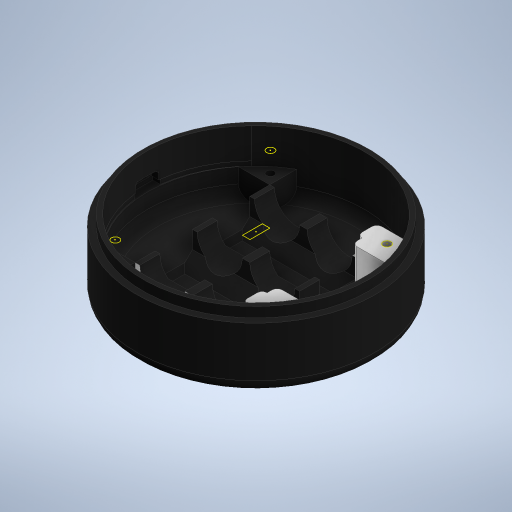
# Autodesk Inventor part: Socle test mesure
Saved by Autodesk Inventor 2024 (Build 280153000, 153)
## iProperties
Created: 2025-01-19
Part Number: Socle test mesure
Material: Générique
Document SubType Name: Modeling
Designer: malam
Density: 1 g/cm^3
Appearance: Par défaut
Author: malam
Autodesk Inventor part; units mm, degrees
ref_plane "YZ Plane" through (0, 0, 0) normal (1, 0, 0) x (0, 1, 0)
ref_plane "XZ Plane" through (0, 0, 0) normal (0, 1, 0) x (-1, 0, 0)
ref_plane "XY Plane" through (0, 0, 0) normal (0, 0, 1) x (1, 0, 0)
sketch "Esquisse1" plane through (0, 0, 0) normal (0, 1, 0) x (-1, 0, 0)
  circle A0 centre (0, 0) radius 45.31
  circle A1 centre (0, 0) radius 47.89
  line L0 (19.5, -32.55) -> (1.5, -32.55)
  line L1 (1.5, -32.55) -> (1.5, 32.55)
  line L2 (1.5, 32.55) -> (19.5, 32.55)
  line L3 (19.5, 32.55) -> (19.5, -32.55)
  line L4 (-1.5, -32.55) -> (-19.5, -32.55)
  line L5 (-19.5, -32.55) -> (-19.5, 32.55)
  line L6 (-19.5, 32.55) -> (-1.5, 32.55)
  line L7 (-1.5, 32.55) -> (-1.5, -32.55)
  line L8 (19.5, -32.55) -> (-19.5, 32.55) construction
  line L9 (19.5, 32.55) -> (-19.5, -32.55) construction
  line L10 (19.5, -32.55) -> (19.5, -43.7402)
  line L11 (19.5, 32.55) -> (19.5, 43.7402)
  point P0 (0, 0)
  point P1 (0, 0)
  dimension "d0" = 90.62
  dimension "d11" = 2.58
  dimension "d16" = 18
  dimension "d17" = 65.1
  dimension "d18" = 18
  dimension "d19" = 3
  constraints: 24 end point, 4 parallel, 2 centre point, 2 horizontal, 2 perpendicular, 2 point on circle, 1 midpoint, 1 point on line, 1 vertical
  measures "d0" diameter of A0
  measures "d11" radial gap between concentric circles of A0 A1
  measures "d16" distance of L1.end L3.start
  measures "d17" distance of L0.end L1.end
  measures "d18" distance of L5.end L7.start
  measures "d19" distance between parallel lines of L7 L1
extrude "Extrusion1" add sketch "Esquisse1" along normal blind 20 contours A0 L11 A1 L10 | A0 L10 A1 L11
sketch "Esquisse4" plane through (0, 0, 0) normal (0, -1, 0) x (1, 0, 0)
  circle A0 centre (0, 0) radius 47.89 projected
  circle A1 centre (0, 0) radius 45.31 projected
extrude "Extrusion4" add sketch "Esquisse4" against normal blind 5 contours A1
fillet "Congé2" radius 5 1 edges at (47.89, 0, 0)
sketch "Esquisse6" plane through (0, 5, 0) normal (0, 1, 0) x (1, 0, 0)
  line L0 (19.5, 32.55) -> (19.5, -32.55) projected
  line L1 (1.5, -32.55) -> (1.5, 32.55) projected
  line L2 (-1.5, 32.55) -> (-1.5, -32.55) projected
  line L3 (-19.5, -32.55) -> (-19.5, 32.55) projected
  line L4 (-19.5, 32.55) -> (-1.5, 32.55) projected
  line L5 (1.5, 32.55) -> (19.5, 32.55) projected
  line L6 (19.5, -32.55) -> (1.5, -32.55) projected
  line L7 (-1.5, -32.55) -> (-19.5, -32.55) projected
  point P0 (0, 0)
sketch "Esquisse7" plane through (0, 20, 0) normal (0, 1, 0) x (1, 0, 0)
  circle A0 centre (0, 0) radius 45.155
  circle A1 centre (0, 0) radius 43.5
  circle A2 centre (0, 0) radius 47.89 projected
  circle A3 centre (0, 0) radius 45.31 projected
  dimension "d35" = 90.31
  dimension "d36" = 87
  constraints: 2 centre point, 2 coincident
  measures "d35" diameter of A0
  measures "d36" diameter of A1
extrude "Extrusion5" add sketch "Esquisse7" against normal up to surface (15 mm away) contours A0 | A3
extrude "Extrusion6" add sketch "Esquisse7" along normal blind 4 contours A0 | A3
ref_plane "Plan de construction1" through (0, 5, 0) normal (0, 1, 0) x (1, 0, 0)
sketch "Esquisse8" plane through (0, 5, 0) normal (0, 1, 0) x (1, 0, 0)
  line L0 (-21.5, -4) -> (21.5, -4)
  line L1 (21.5, -4) -> (21.5, 4)
  line L2 (21.5, 4) -> (-21.5, 4)
  line L3 (-21.5, 4) -> (-21.5, -4)
  line L4 (-21.5, -4) -> (21.5, 4) construction
  line L5 (21.5, -4) -> (-21.5, 4) construction
  line L6 (-21.5, 19) -> (21.5, 19)
  line L7 (21.5, 19) -> (21.5, 27)
  line L8 (21.5, 27) -> (-21.5, 27)
  line L9 (-21.5, 27) -> (-21.5, 19)
  line L10 (-21.5, 19) -> (21.5, 27) construction
  line L11 (21.5, 19) -> (-21.5, 27) construction
  line L12 (-21.5, -27) -> (21.5, -27)
  line L13 (21.5, -27) -> (21.5, -19)
  line L14 (21.5, -19) -> (-21.5, -19)
  line L15 (-21.5, -19) -> (-21.5, -27)
  line L16 (-21.5, -27) -> (21.5, -19) construction
  line L17 (21.5, -27) -> (-21.5, -19) construction
  point P0 (0, 0)
  point P1 (0, 23)
  point P2 (0, -23)
  dimension "d42" = 43
  dimension "d43" = 8
  dimension "d44" = 43
  dimension "d45" = 8
  dimension "d46" = 43
  dimension "d47" = 8
  dimension "d48" = 15
  dimension "d49" = 15
  constraints: 36 end point, 6 midpoint, 6 parallel, 3 horizontal, 3 perpendicular, 2 collinear
  measures "d42" distance of L2.end L1.end
  measures "d43" distance of L0.end L1.end
  measures "d44" distance of L8.end L7.end
  measures "d45" distance of L6.end L7.end
  measures "d46" distance of L14.end L13.end
  measures "d47" distance of L12.end L13.end
  measures "d48" distance between parallel lines of L2 L6
  measures "d49" distance between parallel lines of L14 L0
extrude "Extrusion7" add sketch "Esquisse8" along normal blind 10
sketch "Esquisse9" plane through (-21.5, 5, 27) normal (0, 0, 1) x (1, 0, 0)
  line L0 (43, 0) -> (0, 0) projected
  line L1 (43, 0) -> (43, 10) projected
  line L2 (0, 10) -> (43, 10) projected
  line L3 (0, 0) -> (0, 10) projected
  circle A0 centre (10.95, 10) radius 9.05
  circle A1 centre (32.05, 10) radius 9.05
  point P0 (21.5, -5)
  dimension "d52" = 18.1
  dimension "d53" = 18.1
  dimension "d54" = 21.1
  dimension "d55" = 10.95
  constraints: 2 centre point, 2 point on line
  measures "d52" diameter of A0
  measures "d53" diameter of A1
  measures "d54" distance of A1.centre A0.centre
  measures "d55" distance from line of L3 A0.centre
extrude "Extrusion8" cut sketch "Esquisse9" against normal up to surface (54 mm away) contours A1 L2 | L2 A1 | A0 L2 | L2 A0
sketch "Esquisse10" plane through (0, 5, 0) normal (0, 1, 0) x (1, 0, 0)
  line L0 (22.85, -10.65) -> (38.15, -10.65)
  line L1 (38.15, -10.65) -> (38.15, 10.65)
  line L2 (38.15, 10.65) -> (22.85, 10.65)
  line L3 (22.85, 10.65) -> (22.85, -10.65)
  line L4 (22.85, -10.65) -> (38.15, 10.65) construction
  line L5 (38.15, -10.65) -> (22.85, 10.65) construction
  line L6 (21.5, 19) -> (21.5, 27) projected
  line L7 (21.5, 27) -> (21.5, -27)
  circle A0 centre (0, 0) radius 43.5 projected
  line L8 (21.5, -27) -> (34.1065, -27)
  line L9 (21.5, 27) -> (34.1065, 27)
  line L10 (24.25, -10) -> (36.75, -10)
  line L11 (36.75, -10) -> (36.75, 10)
  line L12 (36.75, 10) -> (24.25, 10)
  line L13 (24.25, 10) -> (24.25, -10)
  line L14 (24.25, -10) -> (36.75, 10) construction
  line L15 (36.75, -10) -> (24.25, 10) construction
  point P0 (30.5, 0)
  dimension "d58" = 15.3
  dimension "d59" = 21.3
  dimension "d60" = 12.5
  dimension "d61" = 20
  dimension "d66" = 9
  constraints: 30 end point, 5 parallel, 4 midpoint, 3 horizontal, 2 perpendicular, 2 point on circle, 1 vertical
  measures "d58" distance of L2.end L1.end
  measures "d59" distance of L1.end L0.end
  measures "d60" distance of L12.end L11.end
  measures "d61" distance of L11.end L10.end
  measures "d66" distance from line of L7 point (30.5, 0)
extrude "Extrusion9" add sketch "Esquisse10" along normal blind 5 contours L3 L2 L1 L0 | L6 L9 A0 L8 L7 picked at (26.1522, -21.55)
extrude "Extrusion10" cut sketch "Esquisse10" against normal up to surface (5 mm away) contours L3 L2 L1 L0 | L13 L12 L11 L10
sketch "Esquisse11" plane through (0, 5, 0) normal (0, -1, 0) x (1, 0, 0)
  line L0 (24.25, 10) -> (36.75, 10) projected
  line L1 (36.75, 10) -> (36.75, -10) projected
  line L2 (36.75, -10) -> (24.25, -10) projected
  line L3 (24.25, -10) -> (24.25, 10) projected
  line L4 (38.15, 10.65) -> (38.15, -10.65) projected
  line L5 (22.85, 10.65) -> (38.15, 10.65) projected
  line L6 (22.85, -10.65) -> (22.85, 10.65) projected
  line L7 (38.15, -10.65) -> (22.85, -10.65) projected
  point P0 (0, 0)
extrude "Extrusion11" cut sketch "Esquisse11" against normal blind 2
sketch "Esquisse12" plane through (0, 20, 0) normal (0, 1, 0) x (1, 0, 0)
  circle A0 centre (0, 0) radius 45.31 projected
  circle A1 centre (0, 0) radius 47.89 projected
extrude "Extrusion12" add sketch "Esquisse12" along normal blind 5
sketch "Esquisse13" plane through (0, 24, 0) normal (0, 1, 0) x (1, 0, 0)
  circle A0 centre (0, 0) radius 45.31 projected
  circle A1 centre (0, 0) radius 43.5 projected
extrude "Extrusion13" add sketch "Esquisse13" along normal blind 5
sketch "Esquisse14" plane through (0, 5, 0) normal (0, 1, 0) x (1, 0, 0)
  line L0 (0, 67.2285) -> (0, -59.7354) construction
  line L1 (0, 0) -> (58.8393, 0) construction
  circle A0 centre (-25.3786, 31.1304) radius 1.35
  circle A1 centre (-25.3786, -31.1304) radius 1.35
  circle A2 centre (0, 0) radius 47.89 construction
  circle A3 centre (0, 0) radius 45.31 construction
  line L2 (-19.6, 27) -> (-21.5, 27) projected
  line L3 (-21.5, 27) -> (-34.1065, 27)
  line L4 (-21.5, 37.8153) -> (-21.5, 27)
  circle A4 centre (0, 0) radius 43.5 projected
  line L5 (-21.5, -27) -> (-34.1065, -27)
  line L6 (-21.5, -37.8153) -> (-21.5, -27)
  constraints: 12 end point, 3 symmetric about line, 2 centre point, 2 horizontal, 2 point on circle, 1 vertical
extrude "Extrusion14" add sketch "Esquisse14" along normal blind 10 contours L3 A4 L4 | L5 L6 A4
sketch "Esquisse15" plane through (0, 15, 0) normal (0, 1, 0) x (1, 0, 0)
  circle A0 centre (-25.3786, 31.1304) radius 1.35 projected
  circle A1 centre (-25.3786, -31.1304) radius 1.35 projected
  circle A2 centre (-25.3786, -31.1304) radius 1.55
  circle A3 centre (-25.3786, 31.1304) radius 1.55
  point P0 (0, 0)
  dimension "d75" = 3.1
  dimension "d76" = 3.1
  constraints: 2 centre point, 2 coincident
  measures "d75" diameter of A2
  measures "d76" diameter of A3
extrude "Extrusion15" cut sketch "Esquisse15" against normal up to surface (10 mm away)
sketch "Esquisse16" plane through (0, 15, 0) normal (0, 1, 0) x (1, 0, 0)
  arc A0 (-45.3383, 4.6099) -> (-45.3383, 4.0099) centre (-45.3383, 4.3099) ccw
  line L0 (-47.6829, 3.1799) -> (-47.6829, 0.4999)
  line L1 (-47.6829, 3.1799) -> (-47.6829, 4.4599)
  line L2 (-45.8829, 4.4599) -> (-47.6829, 4.4599)
  line L3 (-46.4083, 4.9999) -> (-43.3885, 4.9999)
  line L4 (-46.4083, -5.0001) -> (-46.4083, 4.9999)
  line L5 (-47.6829, 0.4899) -> (-47.6829, -3.2001)
  line L6 (-47.6829, -4.4801) -> (-47.6829, -3.2001)
  line L7 (-47.6829, -4.4801) -> (-45.8829, -4.4801)
  line L8 (-43.3885, -5.0001) -> (-46.4083, -5.0001)
  line L9 (-45.3383, -4.0301) -> (-44.5383, -4.0301)
  arc A1 (-45.3383, -4.0301) -> (-45.3383, -4.6301) centre (-45.3383, -4.3301) ccw
  line L10 (-44.5383, -4.6301) -> (-45.3383, -4.6301)
  arc A2 (-44.5383, -4.6301) -> (-44.5383, -4.0301) centre (-44.5383, -4.3301) ccw
  arc A3 (-41.3083, -4.0301) -> (-41.3083, -4.6301) centre (-41.3083, -4.3301) ccw
  line L11 (-41.3083, -4.0301) -> (-40.2083, -4.0301)
  line L12 (-40.2083, -4.6301) -> (-41.3083, -4.6301)
  arc A4 (-27.2104, 33.5062) -> (-43.3885, 4.9999) centre (-1.375, 0) ccw
  line L13 (-44.5383, 4.0099) -> (-45.3383, 4.0099)
  line L14 (-45.3383, 4.6099) -> (-44.5383, 4.6099)
  arc A5 (-44.5383, 4.0099) -> (-44.5383, 4.6099) centre (-44.5383, 4.3099) ccw
  arc A6 (-41.3083, 4.6099) -> (-41.3083, 4.0099) centre (-41.3083, 4.3099) ccw
  line L15 (-40.2083, 4.0099) -> (-41.3083, 4.0099)
  line L16 (-41.3083, 4.6099) -> (-40.2083, 4.6099)
  arc A7 (-40.2083, 4.0099) -> (-40.2083, 4.6099) centre (-40.2083, 4.3099) ccw
  arc A8 (-22.3786, 31.1304) -> (-27.2104, 33.5062) centre (-25.3786, 31.1304) ccw
  circle A9 centre (-25.3786, 31.1303) radius 1.35
  line L17 (-22.3786, 31.1304) -> (-22.3786, -31.1305)
  arc A10 (-27.2104, -33.5063) -> (-22.3786, -31.1305) centre (-25.3786, -31.1305) ccw
  arc A11 (-43.3885, -5.0001) -> (-27.2104, -33.5063) centre (-1.375, -0.0001) ccw
  circle A12 centre (-25.3786, -31.1305) radius 1.35
  arc A13 (-40.2083, -4.6301) -> (-40.2083, -4.0301) centre (-40.2083, -4.3301) ccw
  circle A14 centre (-34.8533, -6.8901) radius 0.5
  circle A15 centre (-32.3133, -6.8901) radius 0.5
  circle A16 centre (-25.3786, 31.1304) radius 1.55 projected
  circle A17 centre (-25.3786, -31.1304) radius 1.55 projected
  circle A18 centre (0, 0) radius 45.31 projected
  circle A19 centre (0, 0) radius 43.5 projected
  circle A20 centre (0, 0) radius 47.89 projected
  circle A21 centre (0, 0) radius 45.31 projected
  line L18 (-43.5657, 5.1999) -> (-46.6083, 5.1999)
  line L19 (-46.6083, 5.1999) -> (-46.6083, -5.2001)
  line L20 (-46.6083, -5.2001) -> (-43.5657, -5.2001)
  arc A22 (-43.5657, -5.2001) -> (-27.3326, -33.6646) centre (-1.375, -0.0001) ccw
  arc A23 (-27.3326, -33.6646) -> (-22.1786, -31.1305) centre (-25.3786, -31.1305) ccw
  line L21 (-22.1786, -31.1305) -> (-22.1786, 31.1304)
  arc A24 (-22.1786, 31.1304) -> (-27.3326, 33.6645) centre (-25.3786, 31.1304) ccw
  arc A25 (-27.3326, 33.6645) -> (-43.5657, 5.1999) centre (-1.375, 0) ccw
  line L22 (-46.6083, 4.6099) -> (-47.6676, 4.6099)
  line L23 (-46.6083, -4.6301) -> (-47.6657, -4.6301)
  point P0 (-31.6526, 29.839)
  point P1 (-31.6504, -29.8413)
  dimension "d79" = 0.2
  constraints: 48 end point, 34 point on circle, 20 centre point, 2 point on line, 1 parallel, 1 perpendicular, 7 other
  measures "d79" radial gap between concentric circles of A4 A25
extrude "Extrusion16" cut sketch "Esquisse16" along normal blind 1.8 contours L14 A18 L13 A0 | A0 L13 A18 L9 A1 L10 L8 L4 L3 L14 | A18 L3 A4 A19 A11 L8 L10 A2 L9 L13 A5 L14 | L14 A5 L13 A18 | A18 L18 A25 A19 A4 L3 | L3 L4 L2 L19 L18 A18 | A18 L10 A1 L9 | L9 A2 L10 A18 | L4 L7 L19 L2 | A18 L20 L19 L7 L4 L8 | L8 A11 A19 A22 L20 A18
sketch "Esquisse18" plane through (0, 15, 0) normal (0, 1, 0) x (1, 0, 0)
  circle A0 centre (-25.3786, 31.1304) radius 1.55 projected
  circle A1 centre (-25.3786, -31.1304) radius 1.55 projected
  line L0 (-21.5, -27) -> (-34.1065, -27) projected
  arc A2 (-34.1065, 27) -> (-34.1065, -27) centre (0, 0) ccw projected
  line L1 (-34.1065, 27) -> (-21.5, 27) projected
  line L2 (-21.5, 27) -> (-21.5, 37.8153) projected
  arc A3 (-21.5, 37.8153) -> (-31.6526, 29.839) centre (0, 0) ccw projected
  arc A4 (-31.6526, 29.839) -> (-43.5657, 5.1999) centre (-1.375, 0) ccw projected
  line L3 (-43.5657, 5.1999) -> (-46.6083, 5.1999) projected
  line L4 (-46.6083, 5.1999) -> (-46.6083, -5.2001) projected
  line L5 (-46.6083, -5.2001) -> (-43.5657, -5.2001) projected
  arc A5 (-43.5657, -5.2001) -> (-31.6504, -29.8413) centre (-1.375, -0.0001) ccw projected
  arc A6 (-31.6504, -29.8413) -> (-21.5, -37.8153) centre (0, 0) ccw projected
  line L6 (-21.5, -37.8153) -> (-21.5, -27) projected
  line L7 (-34.1065, 27) -> (-31.6526, 29.839)
  line L8 (-34.1065, -27) -> (-31.6504, -29.8413)
  arc A7 (-43.5657, 5.1999) -> (-43.5657, -5.2001) centre (-1.3748, -0.0001) ccw
  constraints: 4 end point, 2 point on circle, 1 centre point
extrude "Extrusion17" cut sketch "Esquisse18" along normal through all contours L8 A5 A7 A4 L7 A2
sketch "Esquisse19" plane through (-46.6083, 15, 5.2001) normal (1, 0, 0) x (0, 0, -1)
  line L0 (10.4, 0) -> (0, 0) projected
  line L1 (10.4, 0) -> (10.4, 1.8) projected
  line L2 (10.4, 1.8) -> (0, 1.8) projected
  line L3 (0, 0) -> (0, 1.8) projected
  line L4 (1.58, 5.26) -> (8.82, 5.26)
  line L5 (9.82, 4.26) -> (9.82, 2.8)
  line L6 (8.82, 1.8) -> (1.58, 1.8)
  line L7 (0.58, 2.8) -> (0.58, 4.26)
  line L8 (0.58, 5.26) -> (9.82, 1.8) construction
  line L9 (9.82, 5.26) -> (0.58, 1.8) construction
  arc A0 (1.58, 5.26) -> (0.58, 4.26) centre (1.58, 4.26) ccw
  arc A1 (9.82, 4.26) -> (8.82, 5.26) centre (8.82, 4.26) ccw
  arc A2 (8.82, 1.8) -> (9.82, 2.8) centre (8.82, 2.8) ccw
  arc A3 (0.58, 2.8) -> (1.58, 1.8) centre (1.58, 2.8) ccw
  line L10 (0.58, 2.8) -> (0.58, 1.8)
  line L11 (9.82, 2.8) -> (9.82, 1.8)
  point P0 (5.2001, -15)
  point P1 (5.2, 3.53)
  dimension "d84" = 9.24
  dimension "d85" = 3.46
  dimension "d86" = 1
  dimension "d87" = 1
  dimension "d88" = 0
  constraints: 16 end point, 10 point on line, 10 tangent, 8 point on circle, 4 centre point, 3 perpendicular, 2 equal radius, 2 midpoint, 2 parallel, 1 horizontal
  measures "d84" distance of L8.end L9.end
  measures "d85" distance of L9.start L8.end
  measures "d86" radius of A0
  measures "d87" radius of A1
  measures "d88" distance between parallel lines of L2 L6
extrude "Extrusion18" cut sketch "Esquisse19" against normal blind 15 contours L2 A3 L7 A0 L4 A1 L5 A2
extrude "Extrusion19" cut sketch "Esquisse19" along normal blind 10 contours L2 A2 L11 | L10 A3 L2 | L2 A3 L7 A0 L4 A1 L5 A2
fillet "Congé5" radius 4 3 edges at (8.305, 5, -42.6998) (-43.5, 5, 0) (8.305, 5, 42.6998)
chamfer "Chanfrein2" distance 3 angle 45 4 edges at (0, 5, -19) (0, 5, -4) (0, 5, 4) (0, 5, 19)
chamfer "Chanfrein3" distance 3 angle 45 2 edges at (21.5, 5, -11.5) (21.5, 5, 11.5)
sketch "Esquisse20" plane through (0, 0, 0) normal (0, -1, 0) x (1, 0, 0)
  circle A0 centre (-25, 25) radius 2.5
  circle A1 centre (-25, -25) radius 2.5
  circle A2 centre (25, -25) radius 2.5
  circle A3 centre (25, 25) radius 2.5
  point P0 (0, 0)
  dimension "d103" = 5
  dimension "d104" = 25
  dimension "d105" = 25
  dimension "d108" = 360
  constraints: 4 centre point, 9 other
  measures "d103" diameter of A0
  measures "d104" horizontal distance of point (0, 0) A0.centre
  measures "d105" horizontal distance of point (0, 0) A0.centre
extrude "Extrusion20" cut sketch "Esquisse20" against normal blind 0.5
chamfer "Chanfrein4" distance 2 angle 45 2 edges at (21.5, 10, -11.5) (21.5, 10, 11.5)
sketch "Esquisse21" plane through (0, 5, 0) normal (0, 1, 0) x (1, 0, 0)
  line L0 (18.5, -7) -> (18.5, -16) projected
  line L1 (-21.5, -7) -> (18.5, -7) projected
  line L2 (-21.5, -7) -> (-21.5, 7) projected
  line L3 (18.5, 7) -> (-21.5, 7) projected
  line L4 (18.5, 16) -> (18.5, 7) projected
  line L5 (-21.5, 16) -> (18.5, 16) projected
  line L6 (-21.5, 16) -> (-21.5, 27) projected
  line L7 (-21.5, 27) -> (-28.8314, 27) projected
  arc A0 (-28.8314, 27) -> (-28.8314, -27) centre (0, 0) ccw projected
  line L8 (-28.8314, -27) -> (-21.5, -27) projected
  line L9 (-21.5, -27) -> (-21.5, -16) projected
  line L10 (18.5, -16) -> (-21.5, -16) projected
  line L11 (-21.5, 7) -> (-21.5, 16)
  line L12 (-21.5, -7) -> (-21.5, -16)
  constraints: 4 end point, 1 collinear, 1 vertical
extrude "Extrusion21" cut sketch "Esquisse21" against normal blind 2 contours L0 L10 L12 L1 | L11 L5 L4 L3
chamfer "Chanfrein5" distance 2 angle 45 8 edges at (-21.5, 3, -11.5) (-21.5, 3, 11.5) (18.5, 3, 11.5) (18.5, 3, -11.5) (-1.5, 3, -16) (-1.5, 3, -7) (-1.5, 3, 7) (-1.5, 3, 16)
sketch "Esquisse22" plane through (0, 10, 0) normal (0, 1, 0) x (1, 0, 0)
  line L0 (21.5, -19) -> (23.5, -19) projected
  line L1 (21.5, -27) -> (21.5, -19) projected
  line L2 (21.5, -27) -> (34.1065, -27) projected
  arc A0 (34.1065, -27) -> (34.1065, 27) centre (0, 0) ccw projected
  line L3 (34.1065, 27) -> (21.5, 27) projected
  line L4 (21.5, 19) -> (21.5, 27) projected
  line L5 (23.5, 19) -> (21.5, 19) projected
  line L6 (23.5, 4) -> (23.5, 19) projected
  line L7 (21.5, 4) -> (23.5, 4) projected
  line L8 (21.5, -4) -> (21.5, 4) projected
  line L9 (23.5, -4) -> (21.5, -4) projected
  line L10 (23.5, -19) -> (23.5, -4) projected
  line L11 (24.25, -10) -> (24.25, 10) projected
  line L12 (24.25, 10) -> (36.75, 10) projected
  line L13 (36.75, 10) -> (36.75, -10) projected
  line L14 (36.75, -10) -> (24.25, -10) projected
  line L15 (23.5, 15) -> (40.832, 15)
  line L16 (23.5, -15) -> (40.832, -15)
  circle A1 centre (30.5, 22) radius 1.55
  circle A2 centre (30.5, -22) radius 1.55
  dimension "d120" = 12
  dimension "d121" = 12
  dimension "d122" = 3.1
  dimension "d123" = 5
  dimension "d124" = 9
  dimension "d125" = 3.1
  dimension "d126" = 5
  dimension "d127" = 9
  constraints: 4 end point, 2 centre point, 2 horizontal, 2 point on circle, 2 point on line
  measures "d120" distance between parallel lines of L3 L15
  measures "d121" distance between parallel lines of L2 L16
  measures "d122" diameter of A1
  measures "d123" distance from line of L3 A1.centre
  measures "d124" distance from line of L4 A1.centre
  measures "d125" diameter of A2
  measures "d126" distance from line of L2 A2.centre
  measures "d127" distance from line of L1 A2.centre
extrude "Extrusion22" add sketch "Esquisse22" along normal blind 13 contours L0 L10 L16 A0 L2 L1 | L15 L6 L5 L4 L3 A0
fillet "Congé6" radius 2 6 edges at (23.5, 16.5, -15) (21.5, 19, -19) (21.5, 19, 19) (23.5, 16.5, 15) (21.5, 19, -27) (21.5, 19, 27)
sketch "Esquisse23" plane through (0, 23, 0) normal (0, 1, 0) x (1, 0, 0)
  circle A0 centre (30.5, 22) radius 1.55 projected
  circle A1 centre (30.5, -22) radius 1.55 projected
  line L0 (1.5, -4) -> (1.5, 4) projected
  line L1 (1.5, 4) -> (-1.5, 4) projected
  line L2 (-1.5, 4) -> (-1.5, -4) projected
  line L3 (-1.5, -4) -> (1.5, -4) projected
  circle A2 centre (-25.3786, 31.1304) radius 1.55 projected
  circle A3 centre (-25.3786, -31.1304) radius 1.55 projected
  point P0 (0, 0)
